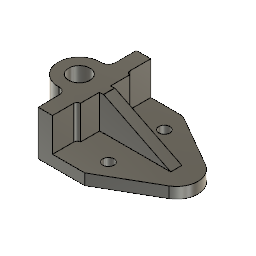
A3 v1 (Autodesk Fusion 360 design; units mm, degrees)
Autodesk Fusion 360 part; units mm, degrees
sketch "Sketch1" plane through (0, 0, 0) normal (0, 0, 1) x (1, 0, 0)
  line L0 (1.7898, -44) -> (-40, -44)
  line L1 (-40, 44) -> (1.7898, 44)
  line L2 (-40, 44) -> (-27, 44)
  line L3 (-27, -44) -> (-40, -44)
  line L4 (-27, 22) -> (-24, 22)
  line L5 (-24, -22) -> (-27, -22)
  line L6 (-24, 5) -> (40, 5)
  line L7 (40, 5) -> (40, -5)
  line L8 (40, -5) -> (-24, -5)
  line L9 (-24, 5) -> (-20, 5)
  line L10 (-20, 5) -> (-20, -5)
  line L11 (-20, -5) -> (-24, -5)
  circle A0 centre (-47, 0) radius 9.5
  circle A1 centre (4, 25) radius 5
  circle A2 centre (4, -25) radius 5
  line L12 (49.5, 16.4545) -> (1.7898, 44)
  line L13 (49.5, -16.4545) -> (1.7898, -44)
  arc A3 (-40, 17.6635) -> (-40, -17.6635) centre (-47, 0) ccw
  line L14 (4.5455, -5) -> (4, -4.4) construction
  line L15 (4, -42.7239) -> (4, -44) construction
  line L16 (4, 5) -> (4, 4.4) construction
  line L17 (4, -4.4) -> (4, -5) construction
  line L18 (4, 4.4) -> (4.5455, 5) construction
  line L19 (-56.5, 0) -> (-59, 0) construction
  line L20 (-20, 0) -> (-27, 0) construction
  line L21 (-37.5, 0) -> (-40, 0) construction
  line L22 (-40, 0) -> (-37.5, 0) construction
  line L23 (-27, 0) -> (-24, 0) construction
  line L24 (40, 5) -> (40, -5)
  arc A4 (49.5, -16.4545) -> (49.5, 16.4545) centre (40, 0) ccw
  line L25 (-24, 22) -> (-24, 5)
  line L26 (-24, -5) -> (-24, -22)
  line L27 (-40, -44) -> (-40, -17.6635)
  line L28 (-40, 17.6635) -> (-40, 44)
  line L29 (-40, -44) -> (-40, -17.6635)
  line L30 (-40, 17.6635) -> (-40, 44)
  line L31 (-27, 44) -> (-27, 22)
  line L32 (-27, -22) -> (-27, -44)
  dimension "d2" = 88
  dimension "d3" = 13
  dimension "d4" = 3
  dimension "d5" = 44
  dimension "d6" = 22
  dimension "d7" = 64
  dimension "d8" = 10
  dimension "d9" = 17
  dimension "d10" = 4
  dimension "d12" = 19
  dimension "d13" = 38
  dimension "d17" = 10
  dimension "d18" = 10
  constraint horizontal L0
  constraint perpendicular L0 L27
  constraint parallel L0 L1
  constraint horizontal L2
  constraint vertical L31
  constraint horizontal L3
  constraint vertical L29
  constraint horizontal L4
  constraint vertical L25
  constraint horizontal L5
  constraint horizontal L6
  constraint vertical L7
  constraint horizontal L8
  constraint horizontal L9
  constraint vertical L10
  constraint horizontal L11
  constraint coincident A0.centre L20
  constraint concentric A0 A3
  constraint coincident A3.start L27
  constraint coincident L23.end L20
  constraint coincident L10 L20.start
  constraint coincident L6 L18.end
  constraint coincident L8 L14.start
  constraint coincident L8 L17.end
  constraint coincident L13 L15.start
  constraint coincident L6 L16.start
  constraint collinear L16 L17
  constraint coincident A0 L19.start
  constraint collinear L19 L20
  constraint coincident L20.end L31
  constraint coincident A0 L21.start
  constraint collinear L20 L21
  constraint collinear L22 L23
  constraint collinear L25 L26
  constraint collinear L27 L28
  constraint collinear L29 L30
  constraint collinear L31 L32
  measures "d2" distance of L0.end L1.start
  measures "d3" distance of L1.start L2.end
  measures "d4" distance of L4.start L4.end
  measures "d5" distance of L4.start L5.end
  measures "d6" distance of L1 L4
  measures "d7" distance of L6.start L6.end
  measures "d8" distance of L6.start L8.end
  measures "d9" distance of L4 L6
  measures "d10" distance of L6.start L9.end
  measures "d12" diameter of A0
  measures "d13" diameter of A3
  measures "d17" diameter of A1
  measures "d18" diameter of A2
extrude "Extrude1" add sketch "Sketch1" along normal blind 10 contours L0 L1 L4 L5 L6 L7 L8 L9 L11 L12 L13 L24 A4 L25 L26 L31 L32
extrude "Extrude2" add sketch "Sketch1" along normal blind 10 contours L6 L7 L8 L10 L24
extrude "Extrude3" add sketch "Sketch1" along normal blind 40 contours L0 L1 L2 L3 L4 L5 L6 L8 L9 L10 L11 A3 L25 L26 L27 L28 L29 L30 L31 L32
fillet "Fillet1" radius 6 1 edges at (-40, -17.6635, 20)
fillet "Fillet2" radius 6 1 edges at (-40, 17.6635, 20)
fillet "Fillet3" radius 3 1 edges at (-27, -22, 25)
fillet "Fillet4" radius 3 1 edges at (-27, 22, 25)
fillet "Fillet5" radius 13 1 edges at (1.7898, 44, 5)
sketch "Sketch2" plane through (0, 0, 0) normal (0, 1, 0) x (1, 0, 0)
  line L0 (39.6527, -10.1952) -> (-20.3473, -10.1952)
  line L1 (-20.3473, -10.1952) -> (-20.3473, -40.1952)
  line L2 (-20.3473, -40.1952) -> (39.6527, -10.1952)
  dimension "d36" = 60
  dimension "d37" = 30
  constraint horizontal L0
  constraint perpendicular L0 L1
  measures "d36" distance of L0.start L0.end
  measures "d37" distance of L0.end L1.end
extrude "Extrude4" add sketch "Sketch2" along normal mid plane 10
equation "d5 = 3 mm + 38 mm + 3 mm"
equation "d7 = 67 mm - 3 mm"
equation "d9 = 14 mm + 3 mm"
equation "d36 = 67 mm - 3 mm - 4 mm"
equation "d37 = 40 mm - 10 mm"
named bodies: "A3"
